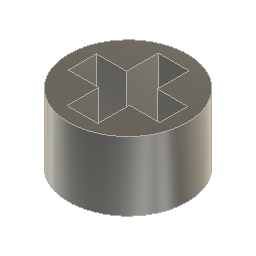
cylindrical_lp_choc_v2 v7 (Autodesk Fusion 360 archive; units mm, degrees)
design "mx_stem"
Autodesk Fusion 360 part; units mm, degrees
sketch "Sketch1" plane through (0, 0, 0) normal (0, 0, 1) x (1, 0, 0)
  line L0 (-0.715, 2.115) -> (0.715, 2.115)
  line L1 (0.715, 2.115) -> (0.715, -2.115)
  line L2 (0.715, -2.115) -> (-0.715, -2.115)
  line L3 (-0.715, -2.115) -> (-0.715, 2.115)
  line L4 (-0.715, 2.115) -> (0.715, -2.115) construction
  line L5 (0.715, 2.115) -> (-0.715, -2.115) construction
  line L6 (-2.115, 0.65) -> (2.115, 0.65)
  line L7 (2.115, 0.65) -> (2.115, -0.65)
  line L8 (2.115, -0.65) -> (-2.115, -0.65)
  line L9 (-2.115, -0.65) -> (-2.115, 0.65)
  line L10 (-2.115, 0.65) -> (2.115, -0.65) construction
  line L11 (2.115, 0.65) -> (-2.115, -0.65) construction
  circle A0 centre (0, 0) radius 2.75
  dimension "d21" = 1.43
  dimension "d22" = 4.23
  dimension "d23" = 4.23
  dimension "d24" = 1.3
  dimension "d25" = 5.5
  constraint horizontal L0
  constraint perpendicular L0 L1
  constraint parallel L0 L2
  constraint parallel L1 L3
  constraint coincident L4 A0.centre
  constraint coincident L5 A0.centre
  constraint coincident A0.centre origin
  constraint horizontal L6
  constraint perpendicular L6 L7
  constraint parallel L6 L8
  constraint parallel L7 L9
  constraint coincident L10 A0.centre
  constraint coincident L11 A0.centre
  measures "d21" distance of L1.end L2.end
  measures "d22" distance of L0.end L1.end
  measures "d23" distance of L7.end L8.end
  measures "d24" distance of L6.end L7.end
  measures "d25" diameter of A0
extrude "Extrude1" add sketch "Sketch1" against normal blind 3.2
chamfer "Chamfer1" distance 0.212 angle 67.02 4 edges at (-2.115, 0, -3.2) (2.115, 0, -3.2) (0, -2.115, -3.2) (0, 2.115, -3.2) measured on face at (-1.6153, -1.0568, -3.2) measured on face at (-1.6153, -1.0568, -3.2) measured on face at (-1.6153, -1.0568, -3.2) measured on face at (-1.6153, -1.0568, -3.2)
chamfer "Chamfer2" distance 0.072 angle 81.8 8 edges at (0.715, 1.4885, -3.2) (1.521, 0.65, -3.2) (1.521, -0.65, -3.2) (0.715, -1.4885, -3.2) (-0.715, -1.4885, -3.2) (-1.521, -0.65, -3.2) (-1.521, 0.65, -3.2) (-0.715, 1.4885, -3.2) measured on face at (-1.0482, 1.709, -3.2) measured on face at (-1.0482, 1.709, -3.2) measured on face at (-1.0482, 1.709, -3.2) measured on face at (-1.0482, 1.709, -3.2) measured on face at (-1.0482, 1.709, -3.2) measured on face at (-1.0482, 1.709, -3.2) measured on face at (-1.0482, 1.709, -3.2) measured on face at (-1.0482, 1.709, -3.2)
equation "width = 5.5 mm"
equation "depth = 5.5 mm"
equation "cross_xy = 4.23 mm"
equation "gap_x = 1.3 mm"
equation "gap_y = 1.43 mm"
equation "height = 3.2 mm" comment "3.7 for mx. 3.3 for choc v2"
equation "d13 = -height"
equation "d15 = chamfer_cross"
equation "d16 = chamfer_cross_angle"
equation "d17 = chamfer_gap"
equation "d18 = chamfer_gap_angle"
equation "d21 = gap_y"
equation "d22 = cross_xy"
equation "d23 = cross_xy"
equation "d24 = gap_x"
equation "d25 = width"
equation "chamfer_cross_angle = 67.02 deg"
equation "chamfer_cross = 0.212 mm"
equation "chamfer_gap_angle = 81.8 deg"
equation "chamfer_gap = 0.072 mm"
